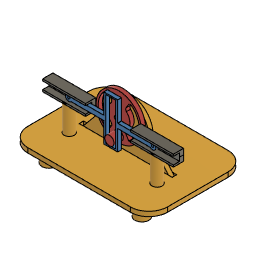
tema numarul 4 primul mecanism facut (Autodesk Fusion 360 design; units mm, degrees)
Autodesk Fusion 360 part; units mm, degrees
sketch "Baza schita" plane through (0, 0, 0) normal (0, 0, 1) x (1, 0, 0) in component "Baza"
  line L0 (149.9987, -105.0118) -> (-150.0016, -105.0118)
  line L1 (149.9984, 104.9886) -> (149.9987, -105.0118)
  line L2 (149.9987, -105.0118) -> (-150.0016, 104.9882) construction
  line L3 (-150.0016, -105.0118) -> (149.9984, 104.9886) construction
  line L4 (49.6882, 4.7) -> (-50.3118, 4.7)
  line L5 (49.6882, -5.0118) -> (-50.3118, -5.0118)
  line L6 (-150.0016, 104.9882) -> (-150.0016, -105.0118)
  line L7 (-150.0016, 104.9882) -> (149.9984, 104.9886)
  line L8 (49.6882, 4.7) -> (49.6882, -5.0118)
  line L9 (-50.3118, 4.7) -> (-50.3118, -5.0118)
  line L10 (-50.3118, -5.0118) -> (-100, -5.0118)
  line L11 (-100, -5.0118) -> (-100, 4.7)
  line L12 (-100, 4.7) -> (-50.3118, 4.7)
  line L13 (49.6882, -5.0118) -> (100, -5.0118)
  line L14 (100, -5.0118) -> (100, 4.7)
  line L15 (100, 4.7) -> (49.6882, 4.7)
  dimension "d1" = 300
  dimension "d2" = 210
  dimension "d11" = 100
  dimension "d12" = 100
  constraint horizontal L0
  constraint horizontal L4
  constraint horizontal L5
  constraint perpendicular L0 L6
  constraint perpendicular L1 L7
  constraint perpendicular L5 L8
  constraint perpendicular L5 L9
  constraint perpendicular L9 L10
  constraint perpendicular L4 L11
  constraint perpendicular L9 L12
  constraint perpendicular L8 L13
  constraint perpendicular L5 L14
  constraint perpendicular L8 L15
  measures "d1" distance of L2.end L1.start
  measures "d2" distance of L0.end L2.end
  measures "d11" distance of L0 L5.end
  measures "d12" distance of L5.start L5.end
extrude "Extrude1" add sketch "Baza schita" along normal blind 10 contours L0 L1 L6 L7 | L4 L5 L8 L9 | L8 L13 L14 L15 | L9 L10 L11 L12 makes body 1 in component "Baza"
sketch "schita suport roata" plane through (0, 0, 0) normal (0, 0, 1) x (1, 0, 0) in component "suport pentru roata"
  line L0 (-100.2047, 5) -> (100.2047, 5)
  line L1 (100.2047, 5) -> (100.2047, -5)
  line L2 (100.2047, -5) -> (-100.2047, -5)
  line L3 (-100.2047, -5) -> (-100.2047, 5)
  constraint horizontal L0
  constraint vertical L1
  constraint horizontal L2
  constraint vertical L3
extrude "Extrude1'" add sketch "Baza schita" along normal blind 110 separate body contours L4 L5 L8 L9 makes body 2 in component "suport pentru roata"
extrude "Extrude2" cut sketch "Baza schita" along normal blind 15 contours L4 L5 L8 L9 bodies 1 in component "Baza"
move_face "OffsetFaces1" offset -0.3 4 faces at (-50.3118, 1.4627, 73.3333) (16.3548, -5.0118, 36.6667) (49.6882, 1.4627, 73.3333) (16.3548, 4.7, 73.3333) on bodies 2 in component "suport pentru roata"
sketch "schita picioruse" plane through (0, 0, 0) normal (0, 0, 1) x (1, 0, 0) in component "picioruse"
  circle A0 centre (-100, -70) radius 15
  circle A1 centre (100, -70) radius 15
  circle A2 centre (-100, 70) radius 15
  circle A3 centre (100, 70) radius 15
  circle A4 centre (-100, 70) radius 15.3
  circle A5 centre (-100, -70) radius 15.3
  circle A6 centre (100, -70) radius 15.3
  circle A7 centre (100, 70) radius 15.3
  circle A8 centre (100, -70) radius 15.3
  line L0 (-150, 105) -> (150, -105) construction
  line L1 (150, 105) -> (-150.0015, -105.0117) construction
  dimension "d22" = 30
  dimension "d26" = 0.3
  dimension "d27" = 0.3
  dimension "d28" = 0.3
  dimension "d29" = 0.3
  dimension "d30" = 0.3
  measures "d22" diameter of A0
extrude "Extrude1''" add sketch "schita picioruse" against normal blind 30 separate body contours A0 | A1 | A2 | A3 makes body 3 at (-85.0745, 68.5065, -20) makes body 4 at (114.9255, 68.5065, -20) makes body 5 at (-85.0745, -71.4935, -20) makes body 6 at (114.9255, -71.4935, -20) in component "picioruse"
extrude "Extrude3" cut sketch "schita picioruse" along normal blind 8 and the other way blind 1 bodies 1 in component "Baza"
extrude "Extrude2'" add sketch "schita picioruse" along normal blind 8 contours A0 | A1 | A2 | A3 bodies 3 4 5 6 in component "picioruse"
sketch "schita pentru mututoi" plane through (0, -4.7118, 0) normal (0, -1, 0) x (1, 0, 0) in component "suport pentru roata"
  line L0 (-50.0118, 0) -> (49.3882, 0)
  line L1 (49.3882, 0) -> (49.3882, 110)
  line L2 (49.3882, 110) -> (-50.0118, 110)
  line L3 (-50.0118, 110) -> (-50.0118, 0)
  line L4 (-50.0118, 110) -> (-50.0118, 10) construction
  line L5 (-50.0118, 10) -> (-50.0118, 90) construction
  circle A0 centre (0, 80) radius 5
  dimension "d37" = 99.4
  dimension "d38" = 100
  dimension "d39" = 80
  dimension "d40" = 10
  constraint coincident L2.end L3.start
  constraint perpendicular L2 L4
  constraint perpendicular L2 L5
  measures "d37" distance of L1.end L2.end
  measures "d38" distance of L2.end L4.end
  measures "d39" distance of L4.end L5.end
  measures "d40" diameter of A0
extrude "Extrude2''" add sketch "schita pentru mututoi" along normal blind 20 separate body contours A0 makes body 7 in component "suport pentru roata"
fillet "Fillet1" radius 40 4 edges at (-150.0016, -105.0118, 5) (149.9987, -105.0118, 5) (149.9984, 104.9886, 5) (-150.0016, 104.9882, 5) on bodies 1 in component "Baza"
fillet "Fillet1'" radius 49.7 2 edges at (49.3882, -0.1559, 110) (-50.0118, -0.1559, 110) on bodies 2 in component "suport pentru roata"
extrude "Extrude4" cut sketch "Baza schita" along normal blind 20 contours L8 L13 L14 L15 | L9 L10 L11 L12 bodies 1 in component "Baza"
sketch "schita2 suport roata" plane through (0, -4.7118, 0) normal (0, -1, 0) x (1, 0, 0) in component "suport pentru roata"
  arc A0 (49.3882, 60.3) -> (-50.0118, 60.3) centre (-0.3118, 60.3) ccw
  line L0 (-50.0118, 60.3) -> (-50.0118, 0)
  line L1 (-50.0118, 0) -> (49.3882, 0)
  line L2 (49.3882, 0) -> (49.3882, 60.3)
  line L3 (49.3882, 60.3) -> (49.3882, 0)
  line L4 (49.3882, 60.3) -> (100, 0)
  line L5 (100, 0) -> (49.3882, 0)
  line L6 (-50.0118, 60.3) -> (-100, 0)
  line L7 (-100, 0) -> (-50.0118, 0)
  line L8 (-50.0118, 60.3) -> (-50.0118, 0)
  constraint coincident A0.start L2.end
  constraint coincident L1.end L2.start
  constraint perpendicular L3 L5
  constraint coincident A0.end L0.start
  constraint coincident L0.end L1.start
  constraint perpendicular L0 L7
extrude "Extrude3'" add sketch "schita2 suport roata" against normal blind 9.112 bodies 7 2 in component "suport pentru roata"
move_face "OffsetFaces2" offset -0.3 2 faces at (-83.3373, 1.3628, 20.1) (83.1294, 1.3628, 20.1) on bodies 7 in component "suport pentru roata"
sketch "schita roata" plane through (0, 0, 0) normal (0, 1, 0) x (1, 0, 0) in component "cerc"
  circle A0 centre (0, -110) radius 5
  circle A1 centre (0, -110) radius 48.5
  dimension "d54" = 10
  dimension "d62" = 97
  constraint concentric A0 A1
  measures "d54" diameter of A0
  measures "d62" diameter of A1
move_face "OffsetFaces3" offset -0.3 1 faces at (4.9938, -18.0452, 79.7508) on bodies 7 in component "suport pentru roata"
extrude "Extrude2'''" add sketch "schita roata" along normal blind -11 and the other way blind 20 separate body makes body 8 in component "cerc"
sketch "schita model roata" plane through (0, 0, 0) normal (0, 1, 0) x (1, 0, 0) in component "cerc"
  circle A0 centre (0, -110) radius 48.5
  spline S0 degree 5 poles (-21.6891, -144.045) (-21.8015, -144.129) (-22.0274, -144.2895) (-22.3696, -144.508) (-22.8328, -144.754) (-23.4241, -144.981) (-24.0286, -145.1207) (-24.6474, -145.1663) (-25.2808, -145.1152) (-25.9282, -144.9722) (-26.5884, -144.7447) (-27.126, -144.5008) (-27.5341, -144.2854) (-27.8083, -144.1275) (-27.946, -144.045) knots 0 0 0 0 0 0 0.1 0.2 0.3 0.4 0.5 0.6 0.7 0.8 0.9 1 1 1 1 1 1
  line L0 (-21.1228, -143.622) -> (-22.2553, -144.468)
  line L1 (-27.3075, -144.4276) -> (-28.5845, -143.6624)
  spline S1 degree 5 poles (-15.4463, -134.2459) (-15.412, -134.1164) (-15.348, -133.8575) (-15.2666, -133.4693) (-15.1873, -132.9521) (-15.1404, -132.3064) (-15.1502, -131.6614) (-15.2212, -131.0173) (-15.3552, -130.374) (-15.5495, -129.7315) (-15.7993, -129.0898) (-16.0397, -128.577) (-16.2415, -128.1927) (-16.3853, -127.9366) (-16.4596, -127.8086) knots 0 0 0 0 0 0 0.1 0.2 0.3 0.4 0.5 0.6 0.7 0.8 0.9 1 1 1 1 1 1
  line L2 (-15.6281, -134.9309) -> (-15.2645, -133.5608)
  line L3 (-16.088, -128.4491) -> (-16.8311, -127.1681)
  spline S2 degree 5 poles (21.6891, -144.045) (21.8015, -144.129) (22.0274, -144.2895) (22.3696, -144.508) (22.8328, -144.754) (23.4241, -144.981) (24.0286, -145.1207) (24.6474, -145.1663) (25.2808, -145.1152) (25.9282, -144.9722) (26.5884, -144.7447) (27.126, -144.5008) (27.5341, -144.2854) (27.8083, -144.1275) (27.946, -144.045) knots 0 0 0 0 0 0 0.1 0.2 0.3 0.4 0.5 0.6 0.7 0.8 0.9 1 1 1 1 1 1
  line L4 (21.1228, -143.622) -> (22.2553, -144.468)
  line L5 (27.3075, -144.4276) -> (28.5845, -143.6624)
  spline S3 degree 5 poles (15.4463, -134.2459) (15.412, -134.1164) (15.348, -133.8575) (15.2666, -133.4693) (15.1873, -132.9521) (15.1404, -132.3064) (15.1502, -131.6614) (15.2212, -131.0173) (15.3552, -130.374) (15.5495, -129.7315) (15.7993, -129.0898) (16.0397, -128.577) (16.2415, -128.1927) (16.3853, -127.9366) (16.4596, -127.8086) knots 0 0 0 0 0 0 0.1 0.2 0.3 0.4 0.5 0.6 0.7 0.8 0.9 1 1 1 1 1 1
  line L6 (15.6281, -134.9309) -> (15.2645, -133.5608)
  line L7 (16.088, -128.4491) -> (16.8311, -127.1681)
  spline S4 degree 5 poles (17.329, -93.0363) (17.2155, -92.9185) (16.9939, -92.682) (16.6782, -92.3249) (16.2909, -91.8437) (15.8668, -91.2335) (15.5084, -90.6136) (15.2214, -89.9831) (15.0098, -89.3416) (14.8715, -88.6892) (14.8016, -88.0268) (14.7961, -87.4895) (14.8185, -87.0825) (14.845, -86.8096) (14.8612, -86.6726) knots 0 0 0 0 0 0 0.1 0.2 0.3 0.4 0.5 0.6 0.7 0.8 0.9 1 1 1 1 1 1
  line L8 (17.9084, -93.6376) -> (16.7496, -92.435)
  line L9 (14.7701, -87.4431) -> (14.9522, -85.9021)
  spline S5 degree 5 poles (28.1197, -76.0983) (27.9659, -76.041) (27.6606, -75.931) (27.209, -75.7798) (26.6198, -75.6064) (25.9066, -75.44) (25.2188, -75.3289) (24.5589, -75.2781) (23.9288, -75.2918) (23.3281, -75.3692) (22.7548, -75.5062) (22.3166, -75.6599) (21.9987, -75.7985) (21.7915, -75.9011) (21.6891, -75.955) knots 0 0 0 0 0 0 0.1 0.2 0.3 0.4 0.5 0.6 0.7 0.8 0.9 1 1 1 1 1 1
  line L10 (28.8237, -76.3608) -> (27.4157, -75.8358)
  line L11 (22.26, -75.6548) -> (21.1182, -76.2551)
  circle A1 centre (0, -75.8521) radius 9.8979
  line L12 (0, -85.75) -> (0, -65.9541)
  spline S6 degree 5 poles (-28.1197, -76.0983) (-27.9659, -76.041) (-27.6606, -75.931) (-27.209, -75.7798) (-26.6198, -75.6064) (-25.9066, -75.44) (-25.2188, -75.3289) (-24.5589, -75.2781) (-23.9288, -75.2918) (-23.3281, -75.3692) (-22.7548, -75.5062) (-22.3166, -75.6599) (-21.9987, -75.7985) (-21.7915, -75.9011) (-21.6891, -75.955) knots 0 0 0 0 0 0 0.1 0.2 0.3 0.4 0.5 0.6 0.7 0.8 0.9 1 1 1 1 1 1
  line L13 (-28.8237, -76.3608) -> (-27.4157, -75.8358)
  line L14 (-22.26, -75.6548) -> (-21.1182, -76.2551)
  spline S7 degree 5 poles (-17.329, -93.0363) (-17.2155, -92.9185) (-16.9939, -92.682) (-16.6782, -92.3249) (-16.2909, -91.8437) (-15.8668, -91.2335) (-15.5084, -90.6136) (-15.2214, -89.9831) (-15.0098, -89.3416) (-14.8715, -88.6892) (-14.8016, -88.0268) (-14.7961, -87.4895) (-14.8185, -87.0825) (-14.845, -86.8096) (-14.8612, -86.6726) knots 0 0 0 0 0 0 0.1 0.2 0.3 0.4 0.5 0.6 0.7 0.8 0.9 1 1 1 1 1 1
  line L15 (-17.9084, -93.6376) -> (-16.7496, -92.435)
  line L16 (-14.7701, -87.4431) -> (-14.9522, -85.9021)
  line L17 (-21.6891, -144.045) -> (-15.4463, -134.2459)
  line L18 (14.8612, -86.6726) -> (21.6891, -75.955)
  line L19 (21.6891, -144.045) -> (15.4463, -134.2459)
  line L20 (-14.8612, -86.6726) -> (-21.6891, -75.955)
  arc A2 (16.4596, -127.8086) -> (17.3282, -93.0355) centre (0, -110) ccw
  arc A3 (-17.3282, -93.0355) -> (-16.4596, -127.8086) centre (0, -110) ccw
  arc A4 (-28.1198, -76.0982) -> (-27.9461, -144.0451) centre (0, -110) ccw
  arc A5 (27.9461, -144.0451) -> (28.1197, -76.0982) centre (0, -110) ccw
  line L21 (-28.1197, -76.0983) -> (-28.1198, -76.0982)
  line L22 (28.1197, -76.0983) -> (28.1197, -76.0982)
  line L23 (27.946, -144.045) -> (27.9461, -144.0451)
  line L24 (-27.946, -144.045) -> (-27.9461, -144.0451)
  point P0 (-24.5675, -145.1417)
  point P1 (-15.2282, -131.0738)
  point P2 (24.5675, -145.1417)
  point P3 (15.2282, -131.0738)
  point P4 (24.3703, -75.2915)
  point P5 (15.2019, -89.8802)
  point P6 (-15.2019, -89.8802)
  point P7 (-24.3703, -75.2915)
  dimension "d65" = 97
  dimension "d67" = 65
  dimension "d76" = 19.7959
  constraint midpoint S0.start L0
  constraint midpoint S0.end L1
  constraint midpoint S1.start L2
  constraint midpoint S1.end L3
  constraint coincident L12.start A1
  constraint midpoint S7.start L15
  constraint midpoint S7.end L16
  constraint midpoint S6.start L13
  constraint midpoint S6.end L14
  constraint collinear L17 L18
  constraint collinear L19 L20
  constraint coincident S7 A3.start
  constraint concentric A2 A3
  constraint coincident S4 A2.end
  constraint concentric A0 A4
  constraint concentric A4 A5
  constraint parallel L19 L23
  measures "d65" diameter of A0
  measures "d67" angle of L17 L19
  measures "d76" distance of L12.start L12.end
extrude "Extrude3''" cut sketch "schita model roata" along normal blind -11 and the other way blind 30 contours S0 S1 S6 S7 L17 L20 A3 A4 | S2 S3 S4 S5 L18 L19 A2 A5 bodies 8 in component "cerc"
extrude "Extrude4'" add sketch "schita model roata" along normal blind -40 and the other way blind 11 contours A1 L12 | A1 L12 bodies 8 in component "cerc"
sketch "mututoi" plane through (0, -40, 0) normal (0, -1, 0) x (1, 0, 0) in component "suport care nu se misca"
  circle A0 centre (0, 75.8521) radius 9.8979
sketch "suport mututoi" plane through (0, -40, 0) normal (0, -1, 0) x (1, 0, 0) in component "suport care nu se misca"
  line L0 (10.64, 64.6903) -> (-10.7259, 64.7208)
  line L1 (-10.7259, 64.7208) -> (-10.5959, 155.7986)
  line L2 (-10.5959, 155.7986) -> (10.6559, 155.7986)
  line L3 (0, 158.5001) -> (15, 158.5001)
  line L4 (15, 158.5001) -> (15, 61.4998)
  line L5 (15, 61.4998) -> (-15, 61.4998)
  line L6 (-15, 61.4998) -> (-15, 158.5001)
  line L7 (-15, 158.5001) -> (0, 158.5001)
  line L8 (10.6559, 155.7986) -> (10.64, 64.6903)
  dimension "d86" = 97.0002
  constraint perpendicular L0 L1
  constraint perpendicular L3 L4
  constraint perpendicular L4 L5
  constraint perpendicular L5 L6
  constraint perpendicular L6 L7
  measures "d86" distance of L5.end L6.end
extrude "Extrude1'''" add sketch "suport mututoi" along normal blind -10 and the other way blind 2 separate body makes body 9 in component "suport care nu se misca"
sketch "BRATE" plane through (15, 0, 0) normal (1, 0, 0) x (0, 1, 0) in component "suport care nu se misca"
  line L0 (-38, 158.5001) -> (-38, 61.4998)
  line L1 (-38, 61.4998) -> (-30, 61.4998)
  line L2 (-30, 61.4998) -> (-30, 158.5001)
  line L3 (-30, 158.5001) -> (-38, 158.5001)
  line L4 (-30, 105) -> (-38, 105)
  line L5 (-38, 105) -> (-38, 115)
  line L6 (-38, 115) -> (-30, 115)
  line L7 (-30, 115) -> (-30, 105)
  dimension "d80" = 10
  dimension "d81" = 10
  constraint horizontal L4
  constraint vertical L5
  constraint horizontal L6
  constraint vertical L7
  constraint coincident L0 L5.end
  constraint coincident L2 L4.start
  measures "d81" distance of L4.end L5.end
extrude "Extrude2''''" add sketch "BRATE" along normal blind 75 and the other way blind 4.344 contours L0 L2 L4 L5 L6 L7 bodies 9 in component "suport care nu se misca"
extrude "Extrude3'''" add sketch "BRATE" along normal blind -105 and the other way blind 26 contours L0 L2 L4 L5 L6 L7 bodies 9 in component "suport care nu se misca"
sketch "CERCULETE" plane through (0, -38, 0) normal (0, -1, 0) x (1, 0, 0) in component "suport care nu se misca"
  line L0 (-15, 105) -> (-15, 61.4998)
  line L1 (-15, 61.4998) -> (15, 61.4998)
  line L2 (15, 61.4998) -> (15, 105)
  line L3 (15, 105) -> (90, 105)
  line L4 (90, 105) -> (90, 115)
  line L5 (90, 115) -> (15, 115)
  line L6 (15, 115) -> (15, 158.5001)
  line L7 (15, 158.5001) -> (-15, 158.5001)
  line L8 (-15, 158.5001) -> (-15, 115)
  line L9 (-15, 115) -> (-90, 115)
  line L10 (-90, 115) -> (-90, 105)
  line L11 (-90, 105) -> (-15, 105)
  line L12 (-10.5959, 155.7986) -> (10.6559, 155.7986)
  line L13 (10.6559, 155.7986) -> (10.64, 64.6903)
  line L14 (10.64, 64.6903) -> (-10.7259, 64.7208)
  line L15 (-10.7259, 64.7208) -> (-10.5959, 155.7986)
  circle A0 centre (-90, 110) radius 2.5
  arc A1 (-85, 115) -> (-85, 105) centre (-90, 110) ccw
  arc A2 (85, 105) -> (85, 115) centre (90, 110) ccw
  circle A3 centre (90, 110) radius 2.5
  dimension "d93" = 5
  dimension "d102" = 30
  constraint concentric A0 A1
  constraint coincident L9 A1.start
  measures "d93" diameter of A0
  measures "d102" distance of L6.end L7.end
extrude "Extrude4''" add sketch "CERCULETE" against normal blind 8 contours L9 L10 L11 A0 A1 | L3 L4 L5 A2 A3 bodies 9 in component "suport care nu se misca"
extrude "Extrude5" cut sketch "CERCULETE" against normal blind 25 contours L10 A0 picked at (-88.5496, 109.6538) bodies 9 in component "suport care nu se misca"
extrude "Extrude6" cut sketch "CERCULETE" against normal blind 40 contours L4 A3 | L4 A3 bodies 9 in component "suport care nu se misca"
sketch "SUPORTI DE SUSTINERE PENTRU SUPORTI" plane through (0, -38, 0) normal (0, -1, 0) x (1, 0, 0) in component "suport care nu se misca"
  circle A0 centre (90, 110) radius 2.5
  circle A1 centre (-90, 110) radius 2.5
  line L0 (85, 115) -> (15, 115)
  line L1 (15, 115) -> (15, 158.5001)
  line L2 (15, 158.5001) -> (-15, 158.5001)
  line L3 (-15, 158.5001) -> (-15, 115)
  line L4 (-15, 115) -> (-85, 115)
  arc A2 (-85, 115) -> (-85, 105) centre (-90, 110) ccw
  line L5 (-85, 105) -> (-15, 105)
  line L6 (-15, 105) -> (-15, 61.4998)
  line L7 (-15, 61.4998) -> (15, 61.4998)
  line L8 (15, 61.4998) -> (15, 105)
  line L9 (15, 105) -> (85, 105)
  arc A3 (85, 105) -> (85, 115) centre (90, 110) ccw
  line L10 (-10.5959, 155.7986) -> (10.6559, 155.7986)
  line L11 (10.6559, 155.7986) -> (10.64, 64.6903)
  line L12 (10.64, 64.6903) -> (-10.7259, 64.7208)
  line L13 (-10.7259, 64.7208) -> (-10.5959, 155.7986)
  line L14 (-140.3586, 121.997) -> (-140.3586, 109.9985)
  line L15 (-140.3586, 109.9985) -> (-48.3586, 109.9985)
  line L16 (-48.3586, 98) -> (-140.3586, 98)
  line L17 (-140.3586, 98) -> (-140.3586, 109.9985)
  line L18 (-48.3586, 121.997) -> (-48.3586, 98)
  line L19 (-140.3586, 118.001) -> (-48.3586, 118.001)
  line L20 (-140.3586, 101.996) -> (-48.3586, 101.996)
  line L21 (-140.3586, 121.997) -> (-48.3586, 121.997)
  line L22 (0, 210) -> (0, 30) construction
  line L23 (140.3586, 121.997) -> (48.3586, 121.997)
  line L24 (48.3586, 121.997) -> (48.3586, 98)
  line L25 (140.3586, 109.9985) -> (48.3586, 109.9985)
  line L26 (140.3586, 118.001) -> (48.3586, 118.001)
  line L27 (140.3586, 101.996) -> (48.3586, 101.996)
  line L28 (48.3586, 98) -> (140.3586, 98)
  line L29 (140.3586, 98) -> (140.3586, 109.9985)
  line L30 (140.3586, 121.997) -> (140.3586, 109.9985)
  dimension "d122" = 92
  dimension "d123" = 92
  constraint vertical L14
  constraint horizontal L15
  constraint symmetric L14.start L15 L16.end
  constraint symmetric L14.end L15 L17.end
  constraint symmetric L15 L19.start L20.start
  constraint vertical L18
  constraint coincident L18 L19.end
  constraint perpendicular L18 L19
  constraint coincident L18 L20.end
  constraint perpendicular L18 L20
  constraint horizontal L21
  constraint parallel L1 L22
  constraint midpoint L15.end L18
  constraint horizontal L16
  constraint coincident L14 L19.start
  constraint symmetric L14.start L22 L23.start
  constraint symmetric L14.end L22 L25.start
  constraint symmetric L15.end L22 L25.end
  constraint symmetric L19.start L22 L26.start
  constraint symmetric L16.start L22 L24.end
  constraint symmetric L16.end L22 L28.end
  constraint symmetric L20.start L22 L27.start
  constraint symmetric L18.start L22 L23.end
  constraint symmetric L19.end L22 L26.end
  constraint symmetric L20.end L22 L27.end
  measures "d122" distance of L14.start L18.start
  measures "d123" distance of L23.start L23.end
extrude "Extrude7" add sketch "SUPORTI DE SUSTINERE PENTRU SUPORTI" along normal blind -17 and the other way blind 8.4 separate body contours A0 L9 A3 L24 L25 | A0 L0 A3 L24 L25 | L9 A3 L24 L25 L27 L29 | L0 A3 L24 L25 L26 L30 | L24 L27 L28 L29 | L23 L24 L26 L30 | A1 L4 A2 L15 L18 | L4 A2 L14 L15 L18 L19 | A2 L5 L15 L17 L18 L20 | A1 A2 L5 L15 L18 | L14 L18 L19 L21 | L16 L17 L18 L20 makes body 10 at (61.4058, -29.6, 109.999) makes body 11 at (-61.4058, -29.6, 109.999) in component "suport care nu se misca"
extrude "Extrude8" add sketch "SUPORTI DE SUSTINERE PENTRU SUPORTI" along normal blind -10 and the other way blind -5 contours L24 L27 L28 L29 | L23 L24 L26 L30 | L14 L18 L19 L21 | L16 L17 L18 L20 bodies 11 10 in component "suport care nu se misca"
extrude "Extrude9" add sketch "SUPORTI DE SUSTINERE PENTRU SUPORTI" along normal blind -17 and the other way blind 8.4 contours A0 L25 | A0 L25 | A1 L15 | A1 L15 bodies 11 10 in component "suport care nu se misca"
sketch "schita suport" plane through (0, 0, 98) normal (0, 0, -1) x (1, 0, 0) in component "picioare suport"
  line L0 (-140.3586, 43) -> (-140.3586, 21)
  line L1 (-140.3586, 21) -> (-48.3586, 21)
  line L2 (-48.3586, 21) -> (-48.3586, 43)
  line L3 (-48.3586, 43) -> (-140.3586, 43)
  line L4 (-140.3586, 43) -> (-48.3586, 21) construction
  line L5 (-48.3586, 43) -> (-140.3586, 21) construction
  line L6 (140.3584, 42.9997) -> (48.3586, 21) construction
  line L7 (140.3584, 21) -> (48.3586, 43) construction
  circle A0 centre (94.3585, 32) radius 10.75
  circle A1 centre (-94.3586, 32) radius 10.75
  dimension "d127" = 21.5
  dimension "d134" = 21.5
  constraint coincident L0.start L3.end
  constraint coincident L1.end L2.start
  constraint coincident L2.end L3.start
  constraint coincident L0.end L1.start
  constraint midpoint L7 A0.centre
  constraint midpoint L5 A1.centre
  measures "d127" diameter of A0
  measures "d134" diameter of A1
sketch "schita gauri pentru suport" plane through (0, 0, 98) normal (0, 0, -1) x (1, 0, 0) in component "suport care nu se misca"
  line L0 (-140.3586, 43) -> (-140.3586, 21)
  line L1 (-140.3586, 21) -> (-48.3586, 21)
  line L2 (-48.3586, 21) -> (-48.3586, 43)
  line L3 (-48.3586, 43) -> (-140.3586, 43)
  line L4 (-140.3586, 43) -> (-48.3586, 21) construction
  line L5 (-48.3586, 43) -> (-140.3586, 21) construction
  circle A0 centre (-94.3586, 32) radius 10.75
  circle A1 centre (-94.3586, 32) radius 10.85
  line L6 (48.3587, 43) -> (140.3587, 43) construction
  line L7 (48.3587, 43) -> (48.3587, 21) construction
  line L8 (48.3587, 21) -> (140.3587, 43) construction
  line L9 (48.3587, 21) -> (140.3587, 21) construction
  line L10 (140.3587, 21) -> (48.3587, 43) construction
  circle A2 centre (94.3587, 32) radius 10.75
  circle A3 centre (94.3587, 32) radius 10.85
  dimension "d137" = 21.5
  dimension "d138" = 0.1
  dimension "d139" = 92
  dimension "d140" = 92
  dimension "d141" = 22
  dimension "d142" = 22
  dimension "d143" = 21.5
  dimension "d144" = 0.1
  constraint coincident L0.start L3.end
  constraint coincident L1.end L2.start
  constraint coincident L2.end L3.start
  constraint coincident L0.end L1.start
  constraint midpoint L4 A0.centre
  constraint perpendicular L2 L6
  constraint perpendicular L6 L7
  constraint perpendicular L7 L9
  constraint midpoint L10 A2.centre
  measures "d137" diameter of A0
  measures "d139" distance of L6.start L6.end
  measures "d140" distance of L0.start L2.end
  measures "d141" distance of L0.start L0.end
  measures "d142" distance of L6.start L7.end
  measures "d143" diameter of A2
extrude "Extrude1''''" add sketch "schita suport" along normal blind 66 and the other way blind 2 separate body contours A0 | A1 makes body 12 at (105.0551, -30.9297, 54) makes body 13 at (-83.6621, -30.9296, 54) in component "picioare suport"
sketch "intrare picioare suporti" plane through (0, 0, 10) normal (0, 0, 1) x (-1, 0, 0) in component "Baza"
  arc A0 (110.0016, -104.9882) -> (150.0016, -64.9882) centre (110.0016, -64.9882) ccw
  line L0 (150.0016, -64.9882) -> (150.0016, 65.0118)
  arc A1 (150.0016, 65.0118) -> (110.0016, 105.0118) centre (110.0016, 65.0118) ccw
  line L1 (110.0016, 105.0118) -> (-109.9987, 105.0118)
  arc A2 (-109.9987, 105.0118) -> (-149.9987, 65.0118) centre (-109.9987, 65.0118) ccw
  line L2 (-149.9987, 65.0118) -> (-149.9985, -64.9886)
  arc A3 (-149.9985, -64.9886) -> (-109.9984, -104.9886) centre (-109.9985, -64.9886) ccw
  line L3 (-109.9984, -104.9886) -> (110.0016, -104.9882)
  line L4 (-100, 5.0118) -> (100, 5.0118)
  line L5 (100, 5.0118) -> (100, -4.7)
  line L6 (100, -4.7) -> (-100, -4.7)
  line L7 (-100, -4.7) -> (-100, 5.0118)
  circle A4 centre (94.3587, 32.0001) radius 10.75
  circle A5 centre (94.3587, 32.0001) radius 11.05
  circle A6 centre (-94.3585, 31.9999) radius 10.75
  circle A7 centre (-94.3585, 31.9999) radius 11.05
  dimension "d128" = 21.5
  dimension "d129" = 0.3
  dimension "d130" = 21.5
  dimension "d131" = 0.3
  measures "d128" diameter of A4
  measures "d130" diameter of A6
extrude "Extrude5'" cut sketch "intrare picioare suporti" against normal blind 8 contours A4 | A5 | A6 | A7 bodies 1 in component "Baza"
sketch "parte sub" plane through (0, 0, 98) normal (0, 0, -1) x (1, 0, 0) in component "suport care nu se misca"
  line L0 (-140.3586, 43) -> (-140.3586, 21)
  line L1 (-140.3586, 21) -> (-48.3586, 21)
  line L2 (-48.3586, 21) -> (-48.3586, 43)
  line L3 (-48.3586, 43) -> (-140.3586, 43)
extrude "Extrude10" cut sketch "schita gauri pentru suport" against normal blind 2 contours A0 | A2 bodies 10 11 in component "suport care nu se misca"
copy_body "Body->Comp2" bodies 9 removing the originals makes body 14 in component "SUPORT MISCATOR"
component "Baza" placed x (1, 0, 0) y (0, 1, 0) z (0, 0, 1) at (0, 0, 30)
component "suport pentru roata" placed x (1, 0, 0) y (0, 1, 0) z (0, 0, 1) at (0, 0, 30)
component "picioruse" placed x (1, 0, 0) y (0, 1, 0) z (0, 0, 1) at (0, 0, 30)
component "cerc" placed x (1, 0, 0) y (0, 1, 0) z (0, 0, 1) at (0, 0, 0)
component "suport care nu se misca" placed x (1, 0, 0) y (0, 1, 0) z (0, 0, 1) at (0, 0, 0)
component "picioare suport" placed x (1, 0, 0) y (0, 1, 0) z (0, 0, 1) at (0, 0, 0)
component "SUPORT MISCATOR" placed x (1, 0, 0) y (0, 1, 0) z (0, 0, 1) at (0, 0, 0)
equation "d87 = -97.00 mm - 30 mm - 5 mm + 27 mm"
named bodies: "suport", "suport roata", "picior spate stg", "picior spate dr", "picior fata stg", "picior fata dr", "roata", "SUPORT MISCATOR", "suport de sustinere 2", "suport sustinere 1", "suport 2", "suport1"
